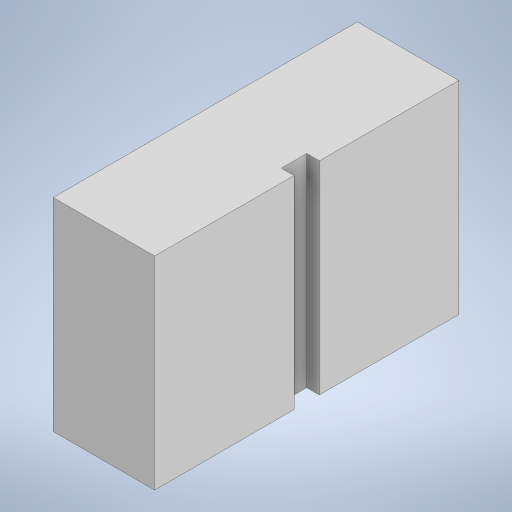
# Autodesk Inventor part: socket_V2
Saved by Autodesk Inventor 2024 (Build 280153000, 153)
## iProperties
Created: 2024-02-20
Part Number: socket_V2
Material: Generic
Document SubType Name: Modeling
Designer: charl
Density: 1 g/cm^3
Appearance: Default
Author: charl
Autodesk Inventor part; units mm, degrees
ref_plane "YZ Plane" through (0, 0, 0) normal (1, 0, 0) x (0, 1, 0)
ref_plane "XZ Plane" through (0, 0, 0) normal (0, 1, 0) x (-1, 0, 0)
ref_plane "XY Plane" through (0, 0, 0) normal (0, 0, 1) x (1, 0, 0)
sketch "Sketch1" plane through (0, 0, 0) normal (0, 1, 0) x (-1, 0, 0)
  line L0 (40, -60) -> (-40, -60)
  line L1 (-40, -60) -> (-40, 60)
  line L2 (-40, 60) -> (40, 60)
  line L3 (40, 60) -> (40, -60)
  line L4 (5, -5) -> (-5, -5)
  line L5 (-5, -5) -> (-5, 5)
  line L6 (-5, 5) -> (5, 5)
  line L7 (5, 5) -> (5, -5)
  point P0 (0, 0)
  point P1 (-5, 0)
  dimension "d1" = 120
  dimension "d2" = 80
  dimension "d3" = 10
  dimension "d4" = 10
  dimension "d5" = 5
  dimension "d6" = 5
  dimension "d7" = 40
  dimension "d8" = 60
  constraints: 16 end point, 4 parallel, 2 horizontal, 2 perpendicular, 1 midpoint
  measures "d1" distance of L2.end L0.start
  measures "d2" distance of L0.start L0.end
  measures "d3" distance of L4.start L4.end
  measures "d4" distance of L6.end L4.start
  measures "d5" distance of point (-5, 0) point (0, 0)
  measures "d6" distance from line of L4 point (0, 0)
  measures "d7" distance from line of L1 point (0, 0)
  measures "d8" distance from line of L0 point (0, 0)
extrude "Extrusion1" add sketch "Sketch1" against normal blind 80
sketch "Sketch5" plane through (40, 0, 60) normal (1, 0, 0) x (0, 0, -1)
  line L0 (120, 0) -> (0, 0) projected
  line L1 (120, 0) -> (120, -80) projected
  line L2 (120, -80) -> (0, -80) projected
  line L3 (0, 0) -> (0, -80) projected
  point P0 (60, 0)
extrude "Extrusion3" cut sketch "Sketch5" against normal blind 40
body "Solid1"
